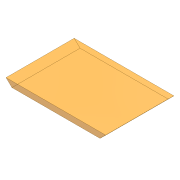
# Autodesk Inventor part: flange7-42mm
Saved by Autodesk Inventor 2021 (Build 250183000, 183)
## iProperties
Created: 2022-10-18
Part Number: flange7-42mm
Material: Rubber, Silicone
Document SubType Name: Modeling
Designer: alyn649
Density: 1.25 g/cm^3
Appearance: Clear - Yellow(1)
Author: alyn649
Autodesk Inventor part; units mm, degrees
ref_plane "YZ Plane" through (0, 0, 0) normal (1, 0, 0) x (0, 1, 0)
ref_plane "XZ Plane" through (0, 0, 0) normal (0, 1, 0) x (-1, 0, 0)
ref_plane "XY Plane" through (0, 0, 0) normal (0, 0, 1) x (1, 0, 0)
sketch "Sketch2" plane through (0, 0, 0) normal (0, 0, 1) x (1, 0, 0)
  line L0 (-13.18, 0) -> (13.18, 0)
  line L1 (13.18, 0) -> (11.6267, -1.5)
  line L2 (11.6267, -1.5) -> (-11.6267, -1.5)
  line L3 (-11.6267, -1.5) -> (-13.18, 0)
  line L4 (-8.8153, 7.7377) -> (-16.0231, 7.7377) construction
  line L5 (13.18, 0) -> (19.7494, 0) construction
  point P0 (0, 0)
  point P1 (0, 0)
  dimension "d0" = 26.36
  dimension "d1" = 136
  dimension "d2" = 136
  dimension "d3" = 1.5
  constraints: 12 end point, 3 horizontal, 1 coincident, 1 midpoint, 1 parallel
  measures "d0" distance of L0.start L0.end
  measures "d1" angle of L3 L4
  measures "d2" angle of L5 L1
  measures "d3" distance between parallel lines of L0 L2
extrude "Extrusion1" add sketch "Sketch2" along normal mid plane 18
equation "\"d2\" = d1"
body "Solid1"
